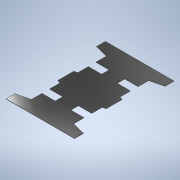
# Autodesk Inventor part: base
Saved by Autodesk Inventor 2021 (Build 250183000, 183)
## iProperties
Created: 2020-10-26
Part Number: base
Material: Generic
Document SubType Name: Modeling
Designer: Mateusz
Density: 1 g/cm^3
Appearance: Default
Author: Mateusz
Autodesk Inventor part; units mm, degrees
ref_plane "YZ Plane" through (0, 0, 0) normal (1, 0, 0) x (0, 1, 0)
ref_plane "XZ Plane" through (0, 0, 0) normal (0, 1, 0) x (-1, 0, 0)
ref_plane "XY Plane" through (0, 0, 0) normal (0, 0, 1) x (1, 0, 0)
sketch "Sketch1" plane through (0, 0, 0) normal (0, 1, 0) x (-1, 0, 0)
  line L0 (359.9997, -324.9998) -> (359.9997, -389.9998)
  line L1 (359.9997, -389.9998) -> (239.9998, -420.0002)
  line L2 (359.9997, -194.9998) -> (359.9997, -129.9998)
  line L3 (359.9997, -129.9998) -> (239.9997, -99.9998)
  line L4 (359.9998, -615.0001) -> (359.9998, -550.0001)
  line L5 (359.9998, -550.0001) -> (239.9998, -520.0001)
  line L6 (359.9998, -745.0001) -> (359.9998, -810.0001)
  line L7 (359.9998, -810.0001) -> (239.9998, -840.0001)
  line L8 (740, -325.0005) -> (740, -390.0005)
  line L9 (740, -390.0005) -> (860, -420.0005)
  line L10 (740, -195.0005) -> (740, -130.0005)
  line L11 (740, -130.0005) -> (860, -100.0005)
  line L12 (740, -615.0001) -> (740, -550.0005)
  line L13 (740, -550.0005) -> (860, -520.0005)
  line L14 (740, -744.9998) -> (740, -809.9998)
  line L15 (740, -809.9998) -> (860, -839.9998)
  line L16 (860, -100.0005) -> (860, -19.9997)
  line L17 (860, -839.9998) -> (860, -919.9998)
  line L18 (239.9997, -99.9998) -> (239.9997, -19.9997)
  line L19 (239.9998, -840.0001) -> (239.9998, -920.0001)
  line L20 (859.9998, -19.9997) -> (379.9998, -19.9997)
  line L21 (860, -19.9997) -> (379.9998, -19.9997)
  line L22 (479.9997, -19.9997) -> (239.9997, -19.9997)
  line L23 (860, -919.9998) -> (139.9998, -919.9998)
  line L24 (239.9997, -19.9997) -> (859.9998, -19.9997)
  line L25 (860, -520.0005) -> (860, -420.0005)
  line L26 (239.9998, -520.0001) -> (239.9998, -420.0002)
  line L27 (479.9998, -744.9997) -> (479.9998, -745.0001)
  line L28 (479.9998, -745.0001) -> (479.9998, -615.0001)
  line L29 (479.9998, -615.0001) -> (359.9998, -615.0001)
  line L30 (479.9998, -745.0001) -> (359.9998, -745.0001)
  line L31 (620, -679.9998) -> (620, -745.0001)
  line L32 (620, -745.0001) -> (740, -744.9998)
  line L33 (620, -679.9998) -> (620, -615.0001)
  line L34 (740, -615.0001) -> (620, -615.0001)
  line L35 (620, -260.0005) -> (620, -325.0005)
  line L36 (620, -325.0005) -> (620, -195.0005)
  line L37 (620, -195.0005) -> (740, -195.0005)
  line L38 (620, -325.0005) -> (740, -325.0005)
  line L39 (479.9997, -260.0005) -> (479.9993, -325.0005)
  line L40 (479.9993, -325.0005) -> (359.9997, -324.9998)
  line L41 (479.9997, -260.0005) -> (479.9997, -195.0005)
  line L42 (479.9997, -195.0005) -> (359.9997, -194.9998)
  point P0 (479.9997, -19.9997)
  point P1 (740, -810.0001)
  point P2 (740, -550.0001)
  point P3 (740, -390.0001)
  point P4 (740, -130.0001)
  point P5 (239.9998, -919.9998)
  point P6 (239.9998, -919.9998)
  dimension "d44" = 0.45
  dimension "d16" = 80
  dimension "d23" = 65
  constraints: 86 end point, 16 point on line, 3 vertical, 2 perpendicular, 1 coincident, 1 horizontal
  measures "d16" distance of L19.end L7.end
  measures "d23" distance of L35.start L35.end
extrude "Extrusion1" add sketch "Sketch1" along normal blind 3
sketch "Sketch2" plane through (0, 3, 0) normal (0, 1, 0) x (1, 0, 0)
  line L0 (-620, 325.0005) -> (-620, 195.0005) projected
  line L1 (-620, 260.0005) -> (-620, 225.0005)
  line L2 (-620, 225.0005) -> (-740, 225.0005)
  line L3 (-740, 195.0005) -> (-740, 130.0005) projected
  line L4 (-740, 225.0005) -> (-740, 195.0005)
  line L5 (-620, 260.0005) -> (-620, 295.0005)
  line L6 (-620, 295.0005) -> (-740, 295.0005)
  line L7 (-740, 295.0005) -> (-740, 325.0005)
  line L8 (-740, 325.0005) -> (-620, 325.0005) projected
  line L9 (-740, 325.0005) -> (-620, 325.0005)
  line L10 (-620, 325.0005) -> (-620, 295.0005)
  line L11 (-620, 225.0005) -> (-620, 195.0005)
  line L12 (-620, 195.0005) -> (-740, 195.0005)
  line L13 (-479.9997, 195.0005) -> (-479.9997, 260.0005) projected
  line L14 (-359.9997, 194.9998) -> (-479.9997, 195.0005) projected
  line L15 (-479.9997, 195.0005) -> (-359.9997, 194.9998)
  line L16 (-359.9997, 194.9998) -> (-359.9995, 225.0005)
  line L17 (-359.9995, 225.0005) -> (-479.9995, 225.0012)
  line L18 (-479.9995, 225.0012) -> (-479.9995, 295.0005)
  line L19 (-479.9997, 260.0005) -> (-479.9993, 325.0005) projected
  line L20 (-479.9993, 325.0005) -> (-359.9997, 324.9998) projected
  line L21 (-479.9993, 325.0005) -> (-359.9997, 324.9998)
  line L22 (-359.9997, 324.9998) -> (-359.9991, 295.0005)
  line L23 (-479.9995, 295.0005) -> (-359.9991, 295.0005)
  line L24 (-620, 745.0001) -> (-620, 615.0001) projected
  line L25 (-620, 680.0001) -> (-620, 645.0001)
  line L26 (-620, 645.0001) -> (-740, 645.0001)
  line L27 (-740, 645.0001) -> (-740, 615.0001)
  line L28 (-740, 615.0001) -> (-620, 615.0001)
  line L29 (-620, 615.0001) -> (-620, 645.0001)
  line L30 (-620, 680.0001) -> (-620, 715.0001)
  line L31 (-620, 715.0001) -> (-740, 715.0001)
  line L32 (-740, 744.9998) -> (-620, 745.0001) projected
  line L33 (-740, 715.0001) -> (-740, 744.9998)
  line L34 (-740, 744.9998) -> (-620, 745.0001)
  line L35 (-620, 745.0001) -> (-620, 715.0001)
  line L36 (-479.9998, 615.0001) -> (-479.9998, 745.0001) projected
  line L37 (-479.9998, 680.0001) -> (-479.9998, 645.0001)
  line L38 (-479.9998, 645.0001) -> (-359.9998, 645.0001)
  line L39 (-359.9998, 615.0001) -> (-479.9998, 615.0001) projected
  line L40 (-359.9998, 645.0001) -> (-359.9998, 615.0001)
  line L41 (-359.9998, 615.0001) -> (-479.9998, 615.0001)
  line L42 (-479.9998, 615.0001) -> (-479.9998, 645.0001)
  line L43 (-479.9998, 680.0001) -> (-479.9998, 715.0001)
  line L44 (-479.9998, 715.0001) -> (-359.9998, 715.0001)
  line L45 (-479.9998, 745.0001) -> (-359.9998, 745.0001) projected
  line L46 (-359.9998, 715.0001) -> (-359.9998, 745.0001)
  line L47 (-359.9998, 745.0001) -> (-479.9998, 745.0001)
  line L48 (-479.9998, 745.0001) -> (-479.9998, 715.0001)
  point P0 (0, 0)
  dimension "d26" = 35
  dimension "d27" = 35
  dimension "d28" = 35
  dimension "d29" = 35
  dimension "d30" = 35
  dimension "d31" = 35
  constraints: 74 end point, 18 perpendicular, 15 point on line, 6 collinear, 3 midpoint
  measures "d26" distance of L1.start L1.end
  measures "d27" distance of L1.start L5.end
  measures "d28" distance of L25.start L25.end
  measures "d29" distance of L25.start L30.end
  measures "d30" distance of L37.start L37.end
  measures "d31" distance of L37.start L43.end
extrude "Extrusion2" add sketch "Sketch2" against normal up to surface (3 mm away)
sketch "Sketch3" plane through (0, 3, 0) normal (0, 1, 0) x (1, 0, 0)
  line L0 (-620, 295.0005) -> (-620, 225.0005) projected
  line L1 (-620, 260.0005) -> (-620, 240.0005)
  line L2 (-620, 240.0005) -> (-479.9995, 240.0005)
  line L3 (-479.9995, 225.0012) -> (-479.9995, 295.0005) projected
  line L4 (-479.9995, 240.0005) -> (-479.9995, 280.0005)
  line L5 (-479.9995, 280.0005) -> (-620, 280.0005)
  line L6 (-620, 280.0005) -> (-620, 260.0005)
  line L7 (-620, 715.0001) -> (-620, 645.0001) projected
  line L8 (-620, 680.0001) -> (-620, 660.0001)
  line L9 (-620, 660.0001) -> (-479.9998, 660.0001)
  line L10 (-479.9998, 645.0001) -> (-479.9998, 715.0001) projected
  line L11 (-479.9998, 660.0001) -> (-479.9998, 680.0001)
  line L12 (-479.9998, 680.0001) -> (-479.9998, 700.0001)
  line L13 (-479.9998, 700.0001) -> (-620, 700.0001)
  line L14 (-620, 700.0001) -> (-620, 680.0001)
  point P0 (0, 0)
  dimension "d34" = 20
  dimension "d35" = 40
  dimension "d36" = 20
  dimension "d37" = 20
  dimension "d38" = 20
  constraints: 22 end point, 7 perpendicular, 7 point on line, 3 midpoint
  measures "d34" distance of L1.start L1.end
  measures "d35" distance of L2.end L4.end
  measures "d36" distance of L8.start L8.end
  measures "d37" distance of L9.end L11.end
  measures "d38" distance of L11.end L12.end
sketch "Sketch4" plane through (0, 3, 0) normal (0, 1, 0) x (1, 0, 0)
  line L0 (-860, 520.0005) -> (-860, 420.0005) projected
  line L1 (-860, 470.0005) -> (-828.2194, 470.0005)
  line L2 (-239.9998, 420.0002) -> (-239.9998, 520.0001) projected
  line L3 (-860, 19.9997) -> (-239.9997, 19.9997) projected
  line L4 (-549.9999, 19.9997) -> (-549.9999, 470.0003)
  line L5 (-549.9999, 470.0003) -> (-549.5499, 470.0003)
  line L6 (-549.9999, 470.0003) -> (-550.4499, 470.0003)
  circle A0 centre (-549.5499, 470.0003) radius 73.409
  point P0 (0, 0)
  dimension "d44" = 0.45
  constraints: 8 end point, 3 horizontal, 2 midpoint, 1 centre point, 1 coincident
  measures "d44" distance of L4.end L5.end
sketch "Sketch7" plane through (0, 3, 0) normal (0, 1, 0) x (1, 0, 0)
  circle A0 centre (-550, 66.9997) radius 3.05
  circle A1 centre (-550, 250.0005) radius 5 projected
  circle A2 centre (-603.85, 270.0005) radius 4.6 projected
  circle A3 centre (-603.85, 250.0005) radius 4.6 projected
  circle A4 centre (-496.15, 250.0005) radius 5 projected
  circle A5 centre (-496.15, 270.0005) radius 5 projected
  line L0 (-537.75, 919.9998) -> (-562.25, 919.9998) projected
  line L1 (-537.75, 879.9998) -> (-537.75, 919.9998) projected
  line L2 (-562.25, 879.9998) -> (-537.75, 879.9998) projected
  line L3 (-562.25, 879.9998) -> (-562.25, 919.9998) projected
  circle A6 centre (-603.85, 690.0001) radius 4.6 projected
  circle A7 centre (-603.85, 670.0001) radius 4.6 projected
  circle A8 centre (-550, 690.0001) radius 4.6 projected
  circle A9 centre (-550, 670.0001) radius 4.6 projected
  circle A10 centre (-496.15, 690.0001) radius 4.6 projected
  circle A11 centre (-496.15, 670.0001) radius 4.6 projected
  circle A12 centre (-550, 66.9997) radius 3
  circle A13 centre (-550, 86.9997) radius 3
  circle A14 centre (-496.15, 250.0005) radius 3
  circle A15 centre (-496.15, 270.0005) radius 3
  circle A16 centre (-550, 250.0005) radius 3
  circle A17 centre (-550, 270.0005) radius 3
  circle A18 centre (-603.85, 250.0005) radius 3
  circle A19 centre (-603.85, 270.0005) radius 3
  circle A20 centre (-496.15, 670.0001) radius 3
  circle A21 centre (-496.15, 690.0001) radius 3
  circle A22 centre (-550, 670.0001) radius 3
  circle A23 centre (-550, 690.0001) radius 3
  circle A24 centre (-603.85, 670.0001) radius 3
  circle A25 centre (-603.85, 690.0001) radius 3
  circle A26 centre (-550, 889.9998) radius 3
  circle A27 centre (-550, 909.9998) radius 3
  point P0 (0, 0)
  dimension "d53" = 6
  dimension "d54" = 6
  dimension "d55" = 6
  dimension "d56" = 6
  dimension "d57" = 6
  dimension "d58" = 6
  dimension "d59" = 6
  dimension "d60" = 6
  dimension "d61" = 6
  dimension "d62" = 6
  dimension "d63" = 6
  dimension "d64" = 6
  dimension "d65" = 6
  dimension "d66" = 6
  dimension "d67" = 6
  dimension "d68" = 6
  constraints: 17 centre point, 12 coincident
  measures "d53" diameter of A12
  measures "d54" diameter of A13
  measures "d55" diameter of A14
  measures "d56" diameter of A15
  measures "d57" diameter of A16
  measures "d58" diameter of A17
  measures "d59" diameter of A18
  measures "d60" diameter of A19
  measures "d61" diameter of A20
  measures "d62" diameter of A21
  measures "d63" diameter of A22
  measures "d64" diameter of A23
  measures "d65" diameter of A24
  measures "d66" diameter of A25
  measures "d67" diameter of A26
  measures "d68" diameter of A27
extrude "Extrusion7" cut sketch "Sketch7" against normal up to surface (3 mm away) contours A12 | A13 | A14 | A15 | A16 | A17 | A18 | A19 | A20 | A21 | A22 | A23 | A24 | A25 | A26 | A27
sketch "Sketch8" plane through (0, 3, 0) normal (0, 1, 0) x (1, 0, 0)
  line L0 (-239.9998, 420.0002) -> (-239.9998, 520.0001) projected
  line L1 (-860, 520.0005) -> (-860, 420.0005) projected
  line L2 (-769.488, 470.0005) -> (-769.488, 542.6285)
  line L3 (-740, 550.0005) -> (-860, 520.0005) projected
  line L4 (-769.488, 470.0005) -> (-769.488, 397.3725)
  line L5 (-860, 420.0005) -> (-740, 390.0005) projected
  line L6 (-330.5118, 470.0001) -> (-330.5118, 542.6281)
  line L7 (-239.9998, 520.0001) -> (-359.9998, 550.0001) projected
  line L8 (-330.5118, 470.0001) -> (-330.5118, 397.3719)
  line L9 (-359.9997, 389.9998) -> (-239.9998, 420.0002) projected
  point P0 (0, 0)
  constraints: 8 end point, 5 point on line, 2 vertical, 1 parallel
extrude "Extrusion8" cut sketch "Sketch8" against normal up to surface (3 mm away)
body "Solid1"
